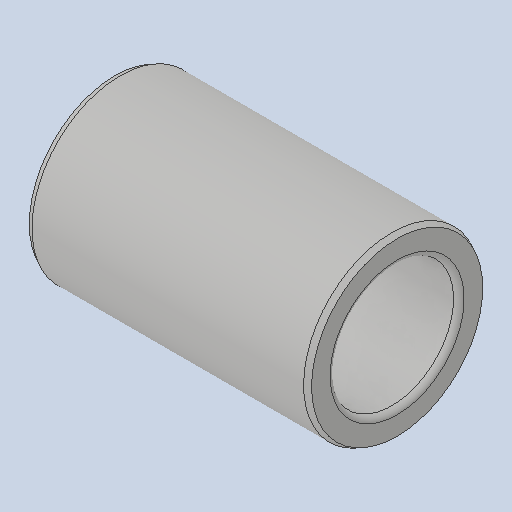
# Autodesk Inventor part: SKF_IR 7X10X16
Saved by Autodesk Inventor 2022 (Build 260153000, 153)
## iProperties
Created: 2022-07-21
Part Number: SKF_IR 7X10X16
Material: Generic
Catalog Web Link: www.cadenas.de
Description: BN1_006-Needle roller bearing inner rings
Vendor: SKF
Document SubType Name: Modeling
Designer: psAdmin
Manufacturer: SKF
Mass: 5 g
Surface Area: 9.21666 cm^2
Volume: 0.63862 cm^3
Density: 1 g/cm^3
Appearance: PSOLRGB-175-175-175
Category: PARTsolutions
Company: SKF
PSOL_IDENT_0: {$CADENAS_DATA/23d-libs/skf/bearings_units_and_housings/roller_bearings/needle_roller_bearings/bn1_0
PSOL_IDENT_1: 06.prj},172 {VTYP=3D},{NB=SKF_IR 7X10X16},{LINA=SKF_IR 7X10X16},{NN=BN1_006},{DATE=08.07.2022 10:25:
PSOL_IDENT_2: 50},{GEOMDATE=31.05.2022 11:15:02},{VERSION=},{LINEID=23890},{WBVAR=},{WBNUMERIC=}  {NB=SKF_IR 7X10X
PSOL_IDENT_3: 16},{LINA=SKF_IR 7X10X16},{KT=DUMMY},{DESIGNATION=IR 7X10X16},{DD=7.000},{F=10.000},{B=16.000},{R12=
PSOL_IDENT_4: 0.300},{HOLE=0.000},{MASS=0.005},{DESIGN=nrb_ir},{IS1=}
NB: SKF_IR 7X10X16
NN: BN1_006
NT: Needle roller bearing inner rings
NBSYN: SKF_$DESIGNATION.
LINA: SKF_IR 7X10X16
CATALOG: SKF
DESIGNATION: IR 7X10X16
DD: 7
F: 10
B: 16
SUPPLIER: SKF
ARTICLENO: SKF_IR 7X10X16
BOMINFO: SKF_IR 7X10X16
CREATOR: CADENAS GmbH
Title: SKF_IR 7X10X16
Author: Cadenas PARTsolutions
Comments: Needle roller bearing inner rings
Autodesk Inventor part; units mm, degrees
ref_plane "YZ Plane" through (0, 0, 0) normal (1, 0, 0) x (0, 1, 0)
ref_plane "XZ Plane" through (0, 0, 0) normal (0, 1, 0) x (-1, 0, 0)
ref_plane "XY Plane" through (0, 0, 0) normal (0, 0, 1) x (1, 0, 0)
sketch "Sketch_1" plane through (0, 0, 0) normal (0, 0, 1) x (1, 0, 0)
  line L0 (50, 0) -> (-50, 0)
  line L1 (0, 4.85) -> (0, 3.8)
  arc A0 (0, 3.8) -> (0.3, 3.5) centre (0.3, 3.8) ccw
  line L2 (0.3, 3.5) -> (15.7, 3.5)
  arc A1 (15.7, 3.5) -> (16, 3.8) centre (15.7, 3.8) ccw
  line L3 (16, 3.8) -> (16, 4.85)
  line L4 (16, 4.85) -> (15.7, 5)
  line L5 (15.7, 5) -> (0.3, 5)
  line L6 (0.3, 5) -> (0, 4.85)
  constraints: 14 end point, 4 point on circle, 2 centre point
revolve "Revolution1" add sketch "Sketch_1" angle 360 about axis through (50, 0, 0) along (1, 0, 0)
body "Solid1"
